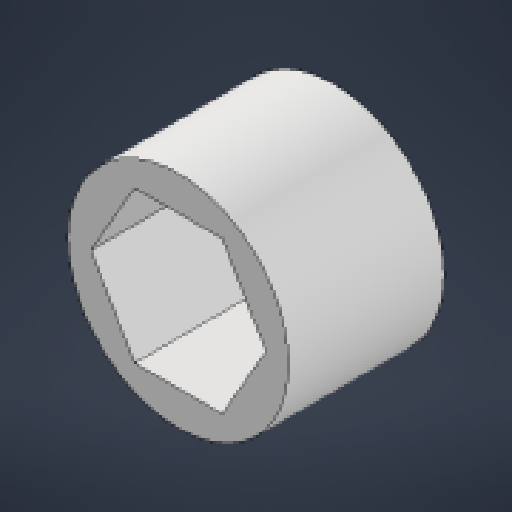
# Autodesk Inventor part: 3DRPINT,FRONT-ROLLER,DRIVE-SPACER
Saved by Autodesk Inventor 2026 (Build 300175000, 175)
## iProperties
Created: 2026-02-10
Part Number: 3DRPINT,FRONT-ROLLER,DRIVE-SPACER
Material: ABS Plastic
Document SubType Name: Modeling
Designer: littl
Density: 1.06 g/cm^3
Appearance: Smooth - White
Author: littl
Autodesk Inventor part; units mm, degrees
ref_plane "YZ Plane" through (0, 0, 0) normal (1, 0, 0) x (0, 1, 0)
ref_plane "XZ Plane" through (0, 0, 0) normal (0, 1, 0) x (-1, 0, 0)
ref_plane "XY Plane" through (0, 0, 0) normal (0, 0, 1) x (1, 0, 0)
sketch "Sketch1" plane through (0, 0, 0) normal (0, 0, 1) x (1, 0, 0)
  line L0 (4.0328, -6.985) -> (-4.0328, -6.985)
  line L1 (-4.0328, -6.985) -> (-8.0656, 0)
  line L2 (-8.0656, 0) -> (-4.0328, 6.985)
  line L3 (-4.0328, 6.985) -> (4.0328, 6.985)
  line L4 (4.0328, 6.985) -> (8.0656, 0)
  line L5 (8.0656, 0) -> (4.0328, -6.985)
  circle A0 centre (0, 0) radius 10.16
  dimension "d0" = 13.97
  dimension "d1" = 20.32
  constraints: 12 end point, 2 coincident, 1 centre point, 1 horizontal, 13 other
  measures "d0" distance between parallel lines of L3 L0
  measures "d1" diameter of A0
extrude "Extrusion1" add sketch "Sketch1" along normal blind 14.2875
body "Solid1"
